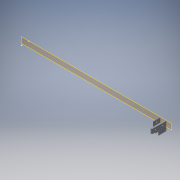
# Autodesk Inventor part: Bed Slider
Saved by Autodesk Inventor 2016 (Build 200138000, 138)
## iProperties
Created: 2016-05-31
Part Number: Bed Slider
Material: Generic
Document SubType Name: Modeling
Designer: Scott
Density: 1 g/cm^3
Appearance: Default
Author: Scott
Autodesk Inventor part; units mm, degrees
ref_plane "YZ Plane" through (0, 0, 0) normal (1, 0, 0) x (0, 1, 0)
ref_plane "XZ Plane" through (0, 0, 0) normal (0, 1, 0) x (-1, 0, 0)
ref_plane "XY Plane" through (0, 0, 0) normal (0, 0, 1) x (1, 0, 0)
ref_plane "Work Plane1" through (0, 0, -304.8) normal (0, 0, 1) x (1, 0, 0)
sketch "Sketch1" plane through (0, 0, -304.8) normal (0, 0, 1) x (1, 0, 0)
  circle A0 centre (602.2484, -36.0888) radius 4 projected
  line L0 (25.4, 0) -> (584.2, 0) projected
  line L1 (584.2, 0) -> (584.2, -20) projected
  line L2 (609.6, -20) -> (584.2, -20) projected
  line L3 (609.6, -20) -> (609.6, 3.175) projected
  line L4 (0, 3.175) -> (609.6, 3.175) projected
  line L5 (0, -20) -> (0, 3.175) projected
  line L6 (25.4, -20) -> (0, -20) projected
  line L7 (25.4, 0) -> (25.4, -20) projected
  circle A1 centre (602.2484, -36.0888) radius 8
  line L8 (595.3202, -40.0888) -> (593.5242, -41.8849)
  line L9 (595.3202, -40.0888) -> (597.8602, -40.0888) construction
  arc A2 (591.8233, -35.0767) -> (612.7225, -36.0888) centre (602.2484, -36.0888) ccw
  line L10 (609.6, -20) -> (584.2, -20)
  line L11 (586.9, -20) -> (606.9, -20)
  line L12 (612.7225, -20) -> (609.6, -20)
  line L13 (612.7225, -36.0888) -> (612.7225, -20)
  line L14 (584.2, -20) -> (591.8233, -35.0767)
  point P0 (0, 0)
  dimension "d0" = 16
  dimension "d1" = 2.54
  dimension "d2" = 135
  dimension "d3" = 20
  constraints: 14 end point, 3 point on circle, 2 coincident, 2 collinear, 1 centre point, 1 equal length, 1 horizontal, 1 point on line, 1 vertical, 3 other
  measures "d1" distance of L8.start L8.end
  measures "d2" angle of L8 L9
  measures "d3" distance of L11.end L11.start
extrude "Extrusion1" add sketch "Sketch1" along normal blind 26 contours L2 L12 L13 A2 L14
sketch "Sketch2" plane through (0, 0, -278.8) normal (0, 0, 1) x (1, 0, 0)
  circle A0 centre (602.2484, -36.0888) radius 8 projected
  line L0 (584.2, -20) -> (591.8233, -35.0767) projected
  arc A1 (591.8233, -35.0767) -> (612.7225, -36.0888) centre (602.2484, -36.0888) ccw projected
  line L1 (612.7225, -36.0888) -> (612.7225, -20) projected
  line L2 (612.7225, -20) -> (584.2, -20) projected
  circle A2 centre (602.2484, -36.0888) radius 6
  point P0 (0, 0)
  dimension "d7" = 12
  constraints: 1 centre point, 1 coincident
  measures "d7" diameter of A2
extrude "Extrusion2" add sketch "Sketch2" along normal blind 2.54 contours A0 | L2 L1 A1 L0
sketch "Sketch3" plane through (0, 0, -304.8) normal (0, 0, -1) x (-1, 0, 0)
  circle A0 centre (-602.2484, -36.0888) radius 6 projected
  line L0 (-584.2, -20) -> (-591.8233, -35.0767) projected
  arc A1 (-612.7225, -36.0888) -> (-591.8233, -35.0767) centre (-602.2484, -36.0888) ccw projected
  line L1 (-612.7225, -36.0888) -> (-612.7225, -20) projected
  line L2 (-612.7225, -20) -> (-584.2, -20) projected
  point P0 (0, 0)
extrude "Extrusion3" add sketch "Sketch3" along normal blind 2.54
sketch "Sketch4" plane through (0, 0, -276.26) normal (0, 0, 1) x (1, 0, 0)
  circle A0 centre (602.2484, -36.0888) radius 6 projected
  line L0 (584.2, -20) -> (591.8233, -35.0767) projected
  arc A1 (591.8233, -35.0767) -> (612.7225, -36.0888) centre (602.2484, -36.0888) ccw projected
  line L1 (612.7225, -36.0888) -> (612.7225, -20) projected
  line L2 (612.7225, -20) -> (584.2, -20) projected
  line L3 (602.2484, -36.0888) -> (610.272, -42.8214)
  arc A2 (591.8233, -35.0767) -> (612.7225, -36.0888) centre (602.2484, -36.0888) ccw projected
  line L4 (602.2484, -36.0888) -> (612.7225, -36.0888) construction
  circle A3 centre (602.2484, -36.0888) radius 6 projected
  line L5 (602.2484, -36.0888) -> (594.2248, -42.8214)
  line L6 (602.2484, -36.0888) -> (612.7225, -36.0888) construction
  arc A4 (594.2248, -42.8214) -> (610.272, -42.8214) centre (602.2484, -36.0888) ccw
  line L7 (602.2484, -36.0888) -> (594.2248, -42.8214)
  line L8 (602.2484, -36.0888) -> (610.272, -42.8214)
  point P0 (0, 0)
  dimension "d12" = 40
  dimension "d13" = 140
  constraints: 12 end point, 4 point on circle, 2 collinear, 2 equal length, 2 horizontal, 1 centre point
  measures "d12" angle of L3 L4
  measures "d13" angle of L5 L6
extrude "Extrusion4" cut sketch "Sketch4" against normal blind 39.0525 contours L5 L3 A0 | A0 L3 A1 L5 picked at (604.1466, -39.5744)
fillet "Fillet1" radius 3.175 2 edges at (596.1201, -41.2311, -291.8) (608.3768, -41.2311, -291.8)
sketch "Sketch5" plane through (0, 0, -276.26) normal (0, 0, 1) x (1, 0, 0)
  point P0 (0, 0)
sketch "Sketch6" plane through (0, 0, -307.34) normal (0, 0, -1) x (-1, 0, 0)
  point P0 (0, 0)
sketch "Sketch7" plane through (0, 0, -307.34) normal (0, 0, -1) x (-1, 0, 0)
  line L0 (-25.4, 0) -> (-584.2, 0) projected
  line L1 (-584.2, 0) -> (-584.2, -20) projected
  line L2 (-609.6, -20) -> (-584.2, -20) projected
  line L3 (-609.6, -20) -> (-609.6, 3.175) projected
  line L4 (0, 3.175) -> (-609.6, 3.175) projected
  line L5 (0, -20) -> (0, 3.175) projected
  line L6 (-25.4, -20) -> (0, -20) projected
  line L7 (-25.4, 0) -> (-25.4, -20) projected
  line L8 (-606.8447, -39.9455) -> (-610.272, -42.8214) projected
  arc A0 (-612.7225, -36.0888) -> (-610.272, -42.8214) centre (-602.2484, -36.0888) ccw projected
  line L9 (-612.7225, -36.0888) -> (-612.7225, -20) projected
  line L10 (-612.7225, -20) -> (-584.2, -20) projected
  line L11 (-584.2, -20) -> (-591.8233, -35.0767) projected
  arc A1 (-594.2248, -42.8214) -> (-591.8233, -35.0767) centre (-602.2484, -36.0888) ccw projected
  line L12 (-594.2248, -42.8214) -> (-597.6521, -39.9455) projected
  arc A2 (-597.6521, -39.9455) -> (-606.8447, -39.9455) centre (-602.2484, -36.0888) ccw projected
  line L13 (-586.4, 0) -> (-586.4, -20)
  line L14 (-607.4, -20) -> (-607.4, 0)
  line L15 (-586.4, 0) -> (-584.2, 0)
  line L16 (-584.2, 0) -> (-584.2, -20)
  line L17 (-584.2, -20) -> (-586.4, -20)
  line L18 (-586.4, 0) -> (-586.4, -20)
  line L19 (-607.4, 0) -> (-609.6, 0)
  line L20 (-609.6, 0) -> (-609.6, -20)
  line L21 (-609.6, -20) -> (-607.4, -20)
  point P0 (0, 0)
  dimension "d17" = 21
  dimension "d18" = 20
  constraints: 18 end point, 2 parallel, 2 perpendicular, 1 collinear, 1 point on line
  measures "d17" distance of L13.end L14.start
  measures "d18" distance of L13.start L13.end
extrude "Extrusion5" add sketch "Sketch7" against normal up to surface (31.08 mm away) contours L1 L2 L13 L15 | L2 L3 L19 L14
sketch "Sketch8" plane through (609.6, -20, -307.34) normal (1, 0, 0) x (0, 0, -1)
  line L0 (-31.08, 20) -> (-31.08, 0) projected
  line L1 (0, 0) -> (-31.08, 0) projected
  line L2 (0, 20) -> (0, 0) projected
  line L3 (0, 20) -> (-31.08, 20) projected
  point P0 (-307.34, 20)
extrude "Extrusion6" add sketch "Sketch8" along normal up to surface (3.1225 mm away)
sketch "Sketch9" plane through (612.7225, -36.0888, -276.26) normal (1, 0, 0) x (0, 0, -1)
  line L0 (0, -3.8567) -> (0, -6.7326) projected
  line L1 (0, -6.7326) -> (0, 0) projected
  line L2 (0, 0) -> (0, 36.0888) projected
  line L3 (0, 16.0888) -> (0, 36.0888) projected
  line L4 (0, 36.0888) -> (0, 16.0888) projected
  line L5 (0, 16.0888) -> (0, 36.0888) projected
  line L6 (0, 16.0888) -> (0, 1.0121) projected
  line L7 (0, 1.0121) -> (0, -6.7326) projected
  line L8 (0, -6.7326) -> (0, -3.8567) projected
  line L9 (0, -3.8567) -> (0, -3.8567) projected
  line L10 (31.08, 16.0888) -> (0, 16.0888) projected
  line L11 (31.08, 16.0888) -> (-32.42, 16.0888)
  line L12 (-32.42, 16.0888) -> (-32.42, 36.0888)
  line L13 (-32.42, 36.0888) -> (31.08, 36.0888)
  line L14 (31.08, 36.0888) -> (31.08, 16.0888)
  point P0 (-276.26, 36.0888)
  dimension "d23" = 63.5
  dimension "d24" = 20
  constraints: 8 end point, 2 parallel, 1 horizontal, 1 perpendicular
  measures "d23" distance of L12.end L13.end
  measures "d24" distance of L11.end L12.end
extrude "Extrusion7" add sketch "Sketch9" against normal up to surface (5.3225 mm away)
sketch "Sketch10" plane through (607.4, -20, -307.34) normal (-1, 0, 0) x (0, 0, 1)
  line L0 (31.08, -16.0888) -> (31.08, 0) projected
  line L1 (0, -16.0888) -> (31.08, -16.0888) projected
  line L2 (0, 20) -> (0, -16.0888) projected
  line L3 (63.5, 20) -> (0, 20) projected
  line L4 (63.5, 20) -> (63.5, 0) projected
  line L5 (63.5, 0) -> (31.08, 0) projected
  circle A0 centre (47.29, 10) radius 2.5
  circle A1 centre (15.54, 10) radius 2.5
  point P0 (307.34, 20)
  dimension "d27" = 5
  dimension "d28" = 5
  constraints: 2 centre point
  measures "d27" diameter of A0
  measures "d28" diameter of A1
extrude "Extrusion8" cut sketch "Sketch10" along normal mid plane 254 contours A0 | A1
body "Solid1"
